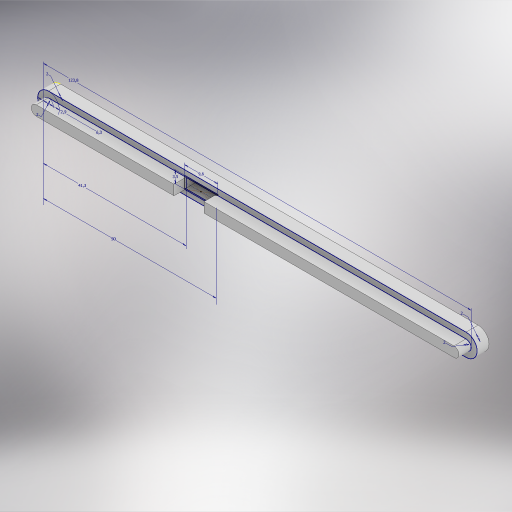
# Autodesk Inventor part: dvddrive-01
Saved by Autodesk Inventor 2024 (Build 280153000, 153)
## iProperties
Created: 2024-08-24
Part Number: dvddrive-01
Material: Generic
Document SubType Name: Modeling
Designer: User
Density: 1 g/cm^3
Appearance: Default
Author: User
Autodesk Inventor part; units mm, degrees
ref_plane "YZ Plane" through (0, 0, 0) normal (1, 0, 0) x (0, 1, 0)
ref_plane "XZ Plane" through (0, 0, 0) normal (0, 1, 0) x (-1, 0, 0)
ref_plane "XY Plane" through (0, 0, 0) normal (0, 0, 1) x (1, 0, 0)
sketch "Sketch1" plane through (0, 0, 0) normal (0, 0, 1) x (1, 0, 0)
  line L0 (0, 0) -> (-120.9, 0) construction
  line L1 (0, 1.45) -> (-120.9, 1.45)
  line L2 (-120.9, -1.45) -> (0, -1.45)
  arc A0 (0, -1.45) -> (0, 1.45) centre (0, 0) ccw
  arc A1 (-120.9, 1.45) -> (-120.9, -1.45) centre (-120.9, 0) ccw
  line L3 (0, 0) -> (-120.9, 0) construction
  line L4 (0, 3.15) -> (-120.9, 3.15)
  line L5 (-120.9, -3.15) -> (0, -3.15)
  arc A2 (0, -3.15) -> (0, 3.15) centre (0, 0) ccw
  arc A3 (-120.9, 3.15) -> (-120.9, -3.15) centre (-120.9, 0) ccw
  line L6 (-72.35, -1.45) -> (-81.05, -1.45)
  line L7 (-81.05, -1.45) -> (-81.05, 1.45)
  line L8 (-81.05, 1.45) -> (-72.35, 1.45)
  line L9 (-72.35, 1.45) -> (-72.35, -1.45)
  line L10 (-71.9, -1.75) -> (-81.5, -1.75)
  line L11 (-81.5, -1.75) -> (-81.5, 1.75)
  line L12 (-81.5, 1.75) -> (-71.9, 1.75)
  line L13 (-71.9, 1.75) -> (-71.9, -1.75)
  line L14 (-71.9, -1.75) -> (-81.5, 1.75) construction
  line L15 (-81.5, -1.75) -> (-71.9, 1.75) construction
  circle A4 centre (0, 0) radius 1
  circle A5 centre (-120.9, 0) radius 1
  point P0 (-60.45, 0)
  point P1 (-122.35, 0)
  point P2 (1.45, 0)
  point P3 (-60.45, 0)
  point P4 (-76.7, 0)
  dimension "d0" = 2.9
  dimension "d1" = 123.8
  dimension "d4" = 6.3
  dimension "d7" = 41.3
  dimension "d8" = 50
  dimension "d9" = 9.6
  dimension "d10" = 3.5
  dimension "d18" = 2
  dimension "d24" = 2
  constraints: 36 end point, 10 point on circle, 8 tangent, 7 parallel, 6 centre point, 4 midpoint, 3 horizontal, 3 point on line, 2 coincident, 2 perpendicular
  measures "d0" diameter of A1
  measures "d1" distance of point (-122.35, 0) point (1.45, 0)
  measures "d4" diameter of A3
  measures "d7" distance from line of point (-122.35, 0) L7
  measures "d8" distance from line of point (-122.35, 0) L9
  measures "d9" distance of L11.end L12.end
  measures "d10" distance of L10.end L11.end
  measures "d18" diameter of A4
  measures "d24" diameter of A5
extrude "Extrusion1" add sketch "Sketch1" along normal blind 3.5 contours L9 L2 L7 L1 | L1 L13 L2 L9 | L7 L2 L11 L1 | L1 A0 L2 L13 | L11 L2 A1 L1 | A4 | A5
extrude "Extrusion2" add sketch "Sketch1" against normal blind 3.5 contours L9 L2 L7 L1 | L1 L11 L12 L13 | L1 L13 L2 L9 | L7 L2 L11 L1 | L1 A0 L2 L13 | L2 L13 L10 L11 | L11 L2 A1 L1 | A2 L5 A3 L4 | A4 | A5
extrude "Extrusion3" cut sketch "Sketch1" along normal blind 3.5 contours L9 L2 L7 L1
extrude "Extrusion4" cut sketch "Sketch1" against normal blind 3.5 contours L9 L2 L7 L1 | L1 L11 L12 L13 | L1 L13 L2 L9 | L7 L2 L11 L1 | L2 L13 L10 L11
chamfer "Chamfer1" distance 0.45 angle 45 2 edges at (-72.35, 0, 0) (-81.05, 0, 0)
sketch "Sketch3" plane through (0, 0, -3.5) normal (0, 0, -1) x (-1, 0, 0)
  arc A0 (120.9, -3.15) -> (120.9, 3.15) centre (120.9, 0) ccw projected
  circle A1 centre (120.9, 0) radius 1
  circle A2 centre (0, 0) radius 1
  dimension "d34" = 2
  dimension "d38" = 2
  constraints: 3 coincident, 2 centre point
  measures "d34" diameter of A1
  measures "d38" diameter of A2
extrude "Extrusion5" [suppressed]
fillet "Fillet2" [suppressed]
fillet "Fillet3" [suppressed]
pattern_linear "Rectangular Pattern1" [suppressed]
extrude "Extrusion6" [suppressed]
fillet "Fillet1" [suppressed]
fillet "Fillet4" [suppressed]
pattern_linear "Rectangular Pattern2" [suppressed]
extrude "Extrusion7" cut sketch "Sketch3" against normal blind 2.5 contours A1
fillet "Fillet5" radius 1 1 edges at (-119.9, 0, -3.5)
extrude "Extrusion8" cut sketch "Sketch3" against normal blind 2.5 contours A2
fillet "Fillet6" radius 1 1 edges at (1, 0, -3.5)
pattern_linear "Rectangular Pattern3" count 12 spacing 6 along (-1, 0, 0) of "Fillet6", "Extrusion8"
pattern_linear "Rectangular Pattern4" count 7 spacing 6 along (1, 0, 0) of "Extrusion7", "Fillet5"
body "Solid1"
